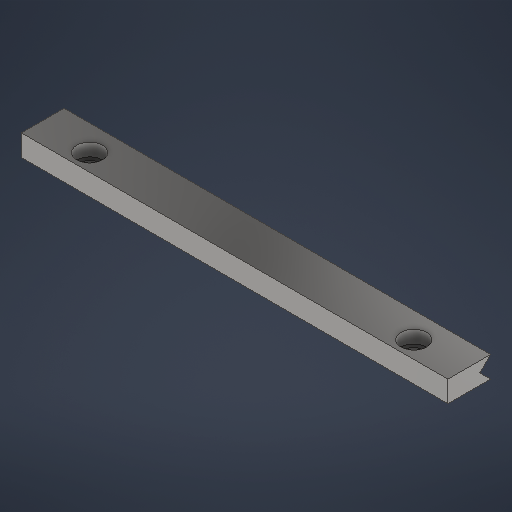
# Autodesk Inventor part: K-tor-kulek
Saved by Autodesk Inventor 2026.1 (Build 301233020, 233B)
## iProperties
Created: 2025-11-03
Part Number: K-tor-kulek
Material: Steel, High Strength, Low Alloy
Document SubType Name: Modeling
Designer: Jan
Density: 7.85 g/cm^3
Appearance: Steel - Polished
Author: Jan
Autodesk Inventor part; units mm, degrees
ref_plane "YZ Plane" through (0, 0, 0) normal (1, 0, 0) x (0, 1, 0)
ref_plane "XZ Plane" through (0, 0, 0) normal (0, 1, 0) x (-1, 0, 0)
ref_plane "XY Plane" through (0, 0, 0) normal (0, 0, 1) x (1, 0, 0)
sketch "Sketch1" plane through (0, 0, 0) normal (1, 0, 0) x (0, 1, 0)
  line L0 (0, 0) -> (5, 0)
  line L1 (5, 0) -> (5, -10)
  line L2 (5, -10) -> (2.5, -7.5)
  line L3 (2.5, -7.5) -> (0, -10)
  line L4 (0, 0) -> (0, -10)
  line L5 (2.5, -7.5) -> (2.5, -12.5) construction
  circle A0 centre (2.5, -10.3284) radius 2 construction
  line L6 (2.5, -10.3284) -> (1.25, -10.3284) construction
  line L7 (5, -10.6569) -> (2.5, -13.1569) construction
  line L8 (2.5, -13.1569) -> (0, -10.6569) construction
  dimension "d0" = 5
  dimension "d3" = 10
  dimension "d4" = 4
  dimension "d33" = 0.6569
  dimension "d34" = 5.6569
  dimension "d35" = 2.8284
  constraints: 18 end point, 3 symmetric about line, 2 horizontal, 2 perpendicular, 2 vertical, 1 centre point, 1 horizontal alignment, 1 parallel, 1 point on line, 1 tangent
  measures "d0" distance of L0.start L0.end
  measures "d3" distance of L0.end L1.end
  measures "d4" diameter of A0
  measures "d33" distance of L7.start L1.end
  measures "d34" distance of L8.start L2.end
  measures "d35" distance of L8.start L6.start
extrude "Extrusion1" add sketch "Sketch1" along normal blind 100
sketch "Sketch2" plane through (0, 5, 0) normal (0, 1, 0) x (1, 0, 0)
  line L0 (0, 10) -> (0, 0) construction
  line L1 (0, 0) -> (100, 0) construction
  line L2 (0, 10) -> (100, 10) construction
  line L3 (12, 0) -> (12, 10) construction
  line L4 (50, 0) -> (50, 15) construction
  circle A0 centre (12, 4) radius 2
  circle A1 centre (88, 4) radius 2
  point P0 (0, 5)
  dimension "d8" = 10
  dimension "d10" = 12
  dimension "d12" = 15
  dimension "d13" = 50
  dimension "d14" = 4
  dimension "d15" = 4
  constraints: 4 end point, 3 point on line, 2 centre point, 2 midpoint, 1 perpendicular, 1 symmetric about line, 1 vertical, 1 other
  measures "d8" distance between parallel lines of L2 L1
  measures "d10" distance from line of L0.end L3
  measures "d12" distance of L4.start L4.end
  measures "d13" distance from line of L0.start L4
  measures "d14" diameter of A0
  measures "d15" vertical distance of L0.end A0.centre
hole "Hole1" at (12, 5, -4) direction (0, -1, 0) diameter 4 end through all counterbore diameter 6 counterbore depth 3
hole "Hole2" at (88, 5, -4) direction (0, -1, 0) diameter 4 end through all counterbore diameter 6 counterbore depth 3
sketch "Sketch3" plane through (100, 0, 0) normal (1, 0, 0) x (0, 0, -1)
  line L0 (0, 5) -> (0, 0) projected
  line L1 (0, 2.5) -> (3, 2.5) construction
  circle A0 centre (3, 2.5) radius 1.6
  dimension "d36" = 3
  dimension "d37" = 3.2
  constraints: 2 end point, 1 centre point, 1 coincident, 1 horizontal, 1 midpoint
  measures "d36" distance of L1.start L1.end
  measures "d37" diameter of A0
hole "Hole3" [suppressed]
chamfer "Chamfer2" [suppressed]
sketch "Sketch4" plane through (0, 0, 0) normal (-1, 0, 0) x (0, 0, 1)
  line L0 (0, 5) -> (0, 0) projected
  circle A0 centre (-3, 2.5) radius 1.7294 projected
  line L1 (0, 2.5) -> (-3, 2.5)
  circle A1 centre (-3, 2.5) radius 1.6
  line L2 (0, 5) -> (0, 0) projected
  dimension "d48" = 3.2
  dimension "d59" = 3
  constraints: 2 end point, 2 midpoint, 1 centre point, 1 coincident, 1 horizontal
  measures "d48" diameter of A1
  measures "d59" distance of point (0, 2.5) L1.end
hole "Hole4" [suppressed]
chamfer "Chamfer3" [suppressed]
body "Solid1"
